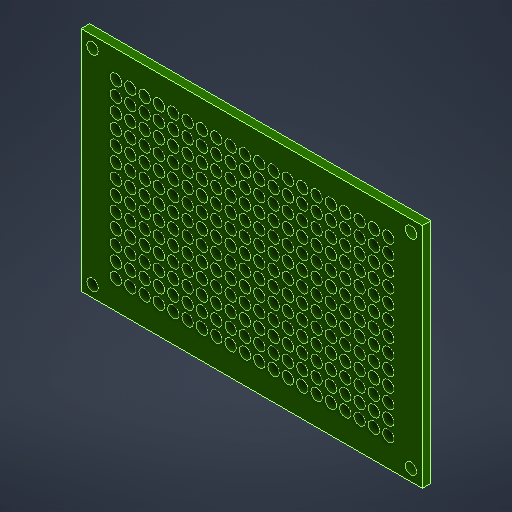
# Autodesk Inventor part: P_PCB_40x60
Saved by Autodesk Inventor 2026 (Build 300175000, 175)
## iProperties
Created: 2025-09-06
Part Number: P_PCB_40x60
Material: Generisch
Document SubType Name: Modeling
Designer: FAL
Density: 1 g/cm^3
Appearance: Vorgabe
Author: FAL
Autodesk Inventor part; units mm, degrees
ref_plane "YZ Plane" through (0, 0, 0) normal (1, 0, 0) x (0, 1, 0)
ref_plane "XZ Plane" through (0, 0, 0) normal (0, 1, 0) x (-1, 0, 0)
ref_plane "XY Plane" through (0, 0, 0) normal (0, 0, 1) x (1, 0, 0)
sketch "Skizze1" plane through (0, 0, 0) normal (0, 1, 0) x (-1, 0, 0)
  line L0 (-30, 20) -> (30, 20)
  line L1 (30, 20) -> (30, -20)
  line L2 (30, -20) -> (-30, -20)
  line L3 (-30, -20) -> (-30, 20)
  line L4 (-30, 20) -> (30, -20) construction
  line L5 (30, 20) -> (-30, -20) construction
  point P0 (0, 0)
  dimension "d0" = 40
  dimension "d1" = 60
  constraints: 12 end point, 2 midpoint, 2 parallel, 1 horizontal, 1 perpendicular
  measures "d0" distance between parallel lines of L2 L0
  measures "d1" distance of L1.end L2.end
extrude "Extrusion1" add sketch "Skizze1" along normal blind 1.5
sketch "Skizze2" plane through (0, 0, 0) normal (0, 1, 0) x (-1, 0, 0)
  line L0 (28, 18) -> (-28, 18) construction
  line L1 (-28, 18) -> (-28, -18) construction
  line L2 (-28, -18) -> (28, -18) construction
  line L3 (28, -18) -> (28, 18) construction
  line L4 (28, 18) -> (-28, -18) construction
  line L5 (-28, 18) -> (28, -18) construction
  circle A0 centre (-28, -18) radius 1
  circle A1 centre (-28, 18) radius 1
  circle A2 centre (28, 18) radius 1
  circle A3 centre (28, -18) radius 1
  point P0 (0, 0)
  dimension "d4" = 36
  dimension "d5" = 56
  dimension "d6" = 2
  constraints: 12 end point, 4 centre point, 4 coincident, 3 equal radius, 2 midpoint, 2 parallel, 1 horizontal, 1 perpendicular
  measures "d4" distance of L2.end L0.start
  measures "d5" distance of L1.end L2.end
  measures "d6" diameter of A0
extrude "Extrusion2" cut sketch "Skizze2" along normal blind 6
sketch "Skizze3" plane through (0, 0, 0) normal (0, 1, 0) x (-1, 0, 0)
  circle A0 centre (-24, -15) radius 1
  line L0 (-30, -20) -> (30, -20) projected
  line L1 (-30, 20) -> (-30, -20) projected
  circle A1 centre (-21.48, -15) radius 1
  circle A2 centre (-18.96, -15) radius 1
  circle A3 centre (-16.44, -15) radius 1
  circle A4 centre (-13.92, -15) radius 1
  circle A5 centre (-11.4, -15) radius 1
  circle A6 centre (-8.88, -15) radius 1
  circle A7 centre (-6.36, -15) radius 1
  circle A8 centre (-3.84, -15) radius 1
  circle A9 centre (-1.32, -15) radius 1
  circle A10 centre (1.2, -15) radius 1
  circle A11 centre (3.72, -15) radius 1
  circle A12 centre (6.24, -15) radius 1
  circle A13 centre (8.76, -15) radius 1
  circle A14 centre (11.28, -15) radius 1
  circle A15 centre (13.8, -15) radius 1
  circle A16 centre (16.32, -15) radius 1
  circle A17 centre (18.84, -15) radius 1
  circle A18 centre (21.36, -15) radius 1
  circle A19 centre (23.88, -15) radius 1
  circle A20 centre (-24, -12.48) radius 1
  circle A21 centre (-21.48, -12.48) radius 1
  circle A22 centre (-18.96, -12.48) radius 1
  circle A23 centre (-16.44, -12.48) radius 1
  circle A24 centre (-13.92, -12.48) radius 1
  circle A25 centre (-11.4, -12.48) radius 1
  circle A26 centre (-8.88, -12.48) radius 1
  circle A27 centre (-6.36, -12.48) radius 1
  circle A28 centre (-3.84, -12.48) radius 1
  circle A29 centre (-1.32, -12.48) radius 1
  circle A30 centre (1.2, -12.48) radius 1
  circle A31 centre (3.72, -12.48) radius 1
  circle A32 centre (6.24, -12.48) radius 1
  circle A33 centre (8.76, -12.48) radius 1
  circle A34 centre (11.28, -12.48) radius 1
  circle A35 centre (13.8, -12.48) radius 1
  circle A36 centre (16.32, -12.48) radius 1
  circle A37 centre (18.84, -12.48) radius 1
  circle A38 centre (21.36, -12.48) radius 1
  circle A39 centre (23.88, -12.48) radius 1
  circle A40 centre (-24, -9.96) radius 1
  circle A41 centre (-21.48, -9.96) radius 1
  circle A42 centre (-18.96, -9.96) radius 1
  circle A43 centre (-16.44, -9.96) radius 1
  circle A44 centre (-13.92, -9.96) radius 1
  circle A45 centre (-11.4, -9.96) radius 1
  circle A46 centre (-8.88, -9.96) radius 1
  circle A47 centre (-6.36, -9.96) radius 1
  circle A48 centre (-3.84, -9.96) radius 1
  circle A49 centre (-1.32, -9.96) radius 1
  circle A50 centre (1.2, -9.96) radius 1
  circle A51 centre (3.72, -9.96) radius 1
  circle A52 centre (6.24, -9.96) radius 1
  circle A53 centre (8.76, -9.96) radius 1
  circle A54 centre (11.28, -9.96) radius 1
  circle A55 centre (13.8, -9.96) radius 1
  circle A56 centre (16.32, -9.96) radius 1
  circle A57 centre (18.84, -9.96) radius 1
  circle A58 centre (21.36, -9.96) radius 1
  circle A59 centre (23.88, -9.96) radius 1
  circle A60 centre (-24, -7.44) radius 1
  circle A61 centre (-21.48, -7.44) radius 1
  circle A62 centre (-18.96, -7.44) radius 1
  circle A63 centre (-16.44, -7.44) radius 1
  circle A64 centre (-13.92, -7.44) radius 1
  circle A65 centre (-11.4, -7.44) radius 1
  circle A66 centre (-8.88, -7.44) radius 1
  circle A67 centre (-6.36, -7.44) radius 1
  circle A68 centre (-3.84, -7.44) radius 1
  circle A69 centre (-1.32, -7.44) radius 1
  circle A70 centre (1.2, -7.44) radius 1
  circle A71 centre (3.72, -7.44) radius 1
  circle A72 centre (6.24, -7.44) radius 1
  circle A73 centre (8.76, -7.44) radius 1
  circle A74 centre (11.28, -7.44) radius 1
  circle A75 centre (13.8, -7.44) radius 1
  circle A76 centre (16.32, -7.44) radius 1
  circle A77 centre (18.84, -7.44) radius 1
  circle A78 centre (21.36, -7.44) radius 1
  circle A79 centre (23.88, -7.44) radius 1
  circle A80 centre (-24, -4.92) radius 1
  circle A81 centre (-21.48, -4.92) radius 1
  circle A82 centre (-18.96, -4.92) radius 1
  circle A83 centre (-16.44, -4.92) radius 1
  circle A84 centre (-13.92, -4.92) radius 1
  circle A85 centre (-11.4, -4.92) radius 1
  circle A86 centre (-8.88, -4.92) radius 1
  circle A87 centre (-6.36, -4.92) radius 1
  circle A88 centre (-3.84, -4.92) radius 1
  circle A89 centre (-1.32, -4.92) radius 1
  circle A90 centre (1.2, -4.92) radius 1
  circle A91 centre (3.72, -4.92) radius 1
  circle A92 centre (6.24, -4.92) radius 1
  circle A93 centre (8.76, -4.92) radius 1
  circle A94 centre (11.28, -4.92) radius 1
  circle A95 centre (13.8, -4.92) radius 1
  circle A96 centre (16.32, -4.92) radius 1
  circle A97 centre (18.84, -4.92) radius 1
  circle A98 centre (21.36, -4.92) radius 1
  circle A99 centre (23.88, -4.92) radius 1
  circle A100 centre (-24, -2.4) radius 1
  circle A101 centre (-21.48, -2.4) radius 1
  circle A102 centre (-18.96, -2.4) radius 1
  circle A103 centre (-16.44, -2.4) radius 1
  circle A104 centre (-13.92, -2.4) radius 1
  circle A105 centre (-11.4, -2.4) radius 1
  circle A106 centre (-8.88, -2.4) radius 1
  circle A107 centre (-6.36, -2.4) radius 1
  circle A108 centre (-3.84, -2.4) radius 1
  circle A109 centre (-1.32, -2.4) radius 1
  circle A110 centre (1.2, -2.4) radius 1
  circle A111 centre (3.72, -2.4) radius 1
  circle A112 centre (6.24, -2.4) radius 1
  circle A113 centre (8.76, -2.4) radius 1
  circle A114 centre (11.28, -2.4) radius 1
  circle A115 centre (13.8, -2.4) radius 1
  circle A116 centre (16.32, -2.4) radius 1
  circle A117 centre (18.84, -2.4) radius 1
  circle A118 centre (21.36, -2.4) radius 1
  circle A119 centre (23.88, -2.4) radius 1
  circle A120 centre (-24, 0.12) radius 1
  circle A121 centre (-21.48, 0.12) radius 1
  circle A122 centre (-18.96, 0.12) radius 1
  circle A123 centre (-16.44, 0.12) radius 1
  circle A124 centre (-13.92, 0.12) radius 1
  circle A125 centre (-11.4, 0.12) radius 1
  circle A126 centre (-8.88, 0.12) radius 1
  circle A127 centre (-6.36, 0.12) radius 1
  circle A128 centre (-3.84, 0.12) radius 1
  circle A129 centre (-1.32, 0.12) radius 1
  circle A130 centre (1.2, 0.12) radius 1
  circle A131 centre (3.72, 0.12) radius 1
  circle A132 centre (6.24, 0.12) radius 1
  circle A133 centre (8.76, 0.12) radius 1
  circle A134 centre (11.28, 0.12) radius 1
  circle A135 centre (13.8, 0.12) radius 1
  circle A136 centre (16.32, 0.12) radius 1
  circle A137 centre (18.84, 0.12) radius 1
  circle A138 centre (21.36, 0.12) radius 1
  circle A139 centre (23.88, 0.12) radius 1
  circle A140 centre (-24, 2.64) radius 1
  circle A141 centre (-21.48, 2.64) radius 1
  circle A142 centre (-18.96, 2.64) radius 1
  circle A143 centre (-16.44, 2.64) radius 1
  circle A144 centre (-13.92, 2.64) radius 1
  circle A145 centre (-11.4, 2.64) radius 1
  circle A146 centre (-8.88, 2.64) radius 1
  circle A147 centre (-6.36, 2.64) radius 1
  circle A148 centre (-3.84, 2.64) radius 1
  circle A149 centre (-1.32, 2.64) radius 1
  circle A150 centre (1.2, 2.64) radius 1
  circle A151 centre (3.72, 2.64) radius 1
  circle A152 centre (6.24, 2.64) radius 1
  circle A153 centre (8.76, 2.64) radius 1
  circle A154 centre (11.28, 2.64) radius 1
  circle A155 centre (13.8, 2.64) radius 1
  circle A156 centre (16.32, 2.64) radius 1
  circle A157 centre (18.84, 2.64) radius 1
  circle A158 centre (21.36, 2.64) radius 1
  circle A159 centre (23.88, 2.64) radius 1
  circle A160 centre (-24, 5.16) radius 1
  circle A161 centre (-21.48, 5.16) radius 1
  circle A162 centre (-18.96, 5.16) radius 1
  circle A163 centre (-16.44, 5.16) radius 1
  circle A164 centre (-13.92, 5.16) radius 1
  circle A165 centre (-11.4, 5.16) radius 1
  circle A166 centre (-8.88, 5.16) radius 1
  circle A167 centre (-6.36, 5.16) radius 1
  circle A168 centre (-3.84, 5.16) radius 1
  circle A169 centre (-1.32, 5.16) radius 1
  circle A170 centre (1.2, 5.16) radius 1
  circle A171 centre (3.72, 5.16) radius 1
  circle A172 centre (6.24, 5.16) radius 1
  circle A173 centre (8.76, 5.16) radius 1
  circle A174 centre (11.28, 5.16) radius 1
  circle A175 centre (13.8, 5.16) radius 1
  circle A176 centre (16.32, 5.16) radius 1
  circle A177 centre (18.84, 5.16) radius 1
  circle A178 centre (21.36, 5.16) radius 1
  circle A179 centre (23.88, 5.16) radius 1
  circle A180 centre (-24, 7.68) radius 1
  circle A181 centre (-21.48, 7.68) radius 1
  circle A182 centre (-18.96, 7.68) radius 1
  circle A183 centre (-16.44, 7.68) radius 1
  circle A184 centre (-13.92, 7.68) radius 1
  circle A185 centre (-11.4, 7.68) radius 1
  circle A186 centre (-8.88, 7.68) radius 1
  circle A187 centre (-6.36, 7.68) radius 1
  circle A188 centre (-3.84, 7.68) radius 1
  circle A189 centre (-1.32, 7.68) radius 1
  circle A190 centre (1.2, 7.68) radius 1
  circle A191 centre (3.72, 7.68) radius 1
  circle A192 centre (6.24, 7.68) radius 1
  circle A193 centre (8.76, 7.68) radius 1
  circle A194 centre (11.28, 7.68) radius 1
  circle A195 centre (13.8, 7.68) radius 1
  circle A196 centre (16.32, 7.68) radius 1
  circle A197 centre (18.84, 7.68) radius 1
  circle A198 centre (21.36, 7.68) radius 1
  circle A199 centre (23.88, 7.68) radius 1
  circle A200 centre (-24, 10.2) radius 1
  circle A201 centre (-21.48, 10.2) radius 1
  circle A202 centre (-18.96, 10.2) radius 1
  circle A203 centre (-16.44, 10.2) radius 1
  circle A204 centre (-13.92, 10.2) radius 1
  circle A205 centre (-11.4, 10.2) radius 1
  circle A206 centre (-8.88, 10.2) radius 1
  circle A207 centre (-6.36, 10.2) radius 1
  circle A208 centre (-3.84, 10.2) radius 1
  circle A209 centre (-1.32, 10.2) radius 1
  circle A210 centre (1.2, 10.2) radius 1
  circle A211 centre (3.72, 10.2) radius 1
  circle A212 centre (6.24, 10.2) radius 1
  circle A213 centre (8.76, 10.2) radius 1
  circle A214 centre (11.28, 10.2) radius 1
  circle A215 centre (13.8, 10.2) radius 1
  circle A216 centre (16.32, 10.2) radius 1
  circle A217 centre (18.84, 10.2) radius 1
  circle A218 centre (21.36, 10.2) radius 1
  circle A219 centre (23.88, 10.2) radius 1
  circle A220 centre (-24, 12.72) radius 1
  circle A221 centre (-21.48, 12.72) radius 1
  circle A222 centre (-18.96, 12.72) radius 1
  circle A223 centre (-16.44, 12.72) radius 1
  circle A224 centre (-13.92, 12.72) radius 1
  circle A225 centre (-11.4, 12.72) radius 1
  circle A226 centre (-8.88, 12.72) radius 1
  circle A227 centre (-6.36, 12.72) radius 1
  circle A228 centre (-3.84, 12.72) radius 1
  circle A229 centre (-1.32, 12.72) radius 1
  circle A230 centre (1.2, 12.72) radius 1
  circle A231 centre (3.72, 12.72) radius 1
  circle A232 centre (6.24, 12.72) radius 1
  circle A233 centre (8.76, 12.72) radius 1
  circle A234 centre (11.28, 12.72) radius 1
  circle A235 centre (13.8, 12.72) radius 1
  circle A236 centre (16.32, 12.72) radius 1
  circle A237 centre (18.84, 12.72) radius 1
  circle A238 centre (21.36, 12.72) radius 1
  circle A239 centre (23.88, 12.72) radius 1
  circle A240 centre (-24, 15.24) radius 1
  circle A241 centre (-21.48, 15.24) radius 1
  circle A242 centre (-18.96, 15.24) radius 1
  circle A243 centre (-16.44, 15.24) radius 1
  circle A244 centre (-13.92, 15.24) radius 1
  circle A245 centre (-11.4, 15.24) radius 1
  circle A246 centre (-8.88, 15.24) radius 1
  circle A247 centre (-6.36, 15.24) radius 1
  circle A248 centre (-3.84, 15.24) radius 1
  circle A249 centre (-1.32, 15.24) radius 1
  circle A250 centre (1.2, 15.24) radius 1
  circle A251 centre (3.72, 15.24) radius 1
  circle A252 centre (6.24, 15.24) radius 1
  circle A253 centre (8.76, 15.24) radius 1
  circle A254 centre (11.28, 15.24) radius 1
  circle A255 centre (13.8, 15.24) radius 1
  circle A256 centre (16.32, 15.24) radius 1
  circle A257 centre (18.84, 15.24) radius 1
  circle A258 centre (21.36, 15.24) radius 1
  circle A259 centre (23.88, 15.24) radius 1
  point P0 (0, 0)
  dimension "d9" = 2
  dimension "d10" = 5
  dimension "d11" = 6
  dimension "d14" = 2.52
  dimension "d17" = 2.52
  constraints: 260 centre point, 1 horizontal, 1 vertical, 518 other
  measures "d9" diameter of A0
  measures "d10" distance from line of L0 A0.centre
  measures "d11" distance from line of L1 A0.centre
  measures "d14" distance of A0.centre A1.centre
  measures "d17" distance of A0.centre A20.centre
extrude "Extrusion3" cut sketch "Skizze3" along normal through all
